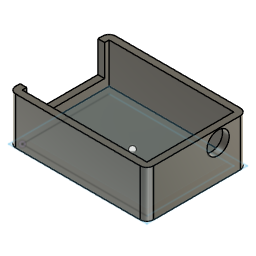
Mini-Amp Case (Autodesk Fusion 360 design; units mm, degrees)
Autodesk Fusion 360 part; units mm, degrees
sketch "Sketch1" plane through (0, 0, 0) normal (0, 0, 1) x (1, 0, 0)
  line L0 (0, 0) -> (56, 0)
  line L1 (56, 0) -> (56, 39)
  line L2 (56, 39) -> (0, 39)
  line L3 (0, 39) -> (0, 0)
  line L4 (-3, -3) -> (59, -3)
  line L5 (59, -3) -> (59, 42)
  line L6 (59, 42) -> (-3, 42)
  line L7 (-3, 42) -> (-3, -3)
  constraint horizontal L0
  constraint vertical L1
  constraint horizontal L2
  constraint vertical L3
  constraint coincident L0.start L3.end
  constraint horizontal L4
  constraint vertical L5
  constraint horizontal L6
  constraint vertical L7
extrude "Extrude1" add sketch "Sketch1" along normal blind 3 contours L0 L1 L2 L3 | L4 L5 L6 L7
extrude "Extrude2" add sketch "Sketch1" along normal blind 21
sketch "Sketch2" plane through (59, 0, 0) normal (1, 0, 0) x (0, 1, 0)
  line L0 (-3, 0) -> (42, 0)
  line L1 (42, 0) -> (42, 21)
  line L2 (42, 21) -> (-3, 21)
  line L3 (-3, 21) -> (-3, 0)
  line L4 (42, 0) -> (42, 15.5) construction
  line L5 (42, 15.5) -> (29, 15.5) construction
  circle A0 centre (29, 15.5) radius 5
  constraint coincident L0.end L1.start
  constraint coincident L1 L4.end
  constraint perpendicular L0 L4
  constraint perpendicular L4 L5
  constraint coincident L5.end A0.centre
extrude "Extrude3" cut sketch "Sketch2" against normal blind 3 contours A0
sketch "Sketch3" plane through (-3, 0, 0) normal (-1, 0, 0) x (0, -1, 0)
  line L0 (-42, 0) -> (3, 0)
  line L1 (3, 0) -> (3, 21)
  line L2 (3, 21) -> (-42, 21)
  line L3 (-42, 21) -> (-42, 0)
  line L4 (-37, 7) -> (-37, 21)
  line L5 (-37, 21) -> (-2, 21)
  line L6 (-2, 21) -> (-2, 7)
  line L7 (-2, 7) -> (-37, 7)
  constraint perpendicular L0 L4
  constraint perpendicular L1 L5
  constraint perpendicular L5 L6
  constraint perpendicular L4 L7
  constraint coincident L2 L4.end
extrude "Extrude4" cut sketch "Sketch3" against normal blind 3 contours L2 L4 L5 L6 L7
fillet "Fillet1" radius 3 4 edges at (59, -3, 10.5) (59, 42, 10.5) (-3, 42, 10.5) (-3, -3, 10.5)
sketch "Sketch4" plane through (0, 0, 3) normal (0, 0, 1) x (-1, 0, 0)
  line L0 (0, 0) -> (-56, 0)
  line L1 (-56, 0) -> (-56, -39)
  line L2 (-56, -39) -> (0, -39)
  line L3 (0, -39) -> (0, 0)
  point P0 (-29.8405, -19.6761)
